Autodesk Fusion 360 part; units mm, degrees
note: some values were not read from the file. Set by a fixed rule: which sketch regions a step uses.
(part 8 of 15)
  line L6133 (281.912, -140.435) -> (281.972, -140.711)
  line L6134 (55.3535, -142.69) -> (55.0989, -142.813)
  line L6135 (56.3211, -141.359) -> (56.2444, -141.631)
  line L6136 (274.039, -141.862) -> (274.06, -141.678)
  line L6137 (56.1301, -141.889) -> (55.9807, -142.129)
  line L6138 (52.4255, -141.451) -> (52.3747, -141.173)
  line L6139 (52.6411, -141.971) -> (52.5149, -141.719)
  line L6140 (275.765, -142.423) -> (275.644, -142.563)
  line L6141 (52.5666, -140.073) -> (52.7085, -139.829)
  line L6142 (53.8349, -139.024) -> (54.112, -138.969)
  line L6143 (53.4546, -142.735) -> (53.2126, -142.589)
  line L6144 (56.3427, -140.671) -> (56.3626, -140.953)
  line L6145 (275.644, -142.563) -> (275.498, -142.677)
  line L6146 (275.52, -141.088) -> (275.663, -141.206)
  line L6147 (274.785, -142.803) -> (274.609, -142.746)
  line L6148 (52.4605, -140.335) -> (52.5666, -140.073)
  line L6149 (274.609, -142.746) -> (274.447, -142.655)
  line L6150 (274.447, -142.655) -> (274.306, -142.535)
  line L6151 (53.2126, -142.589) -> (52.9935, -142.411)
  line L6152 (56.2832, -140.395) -> (56.3427, -140.671)
  line L6153 (274.055, -142.047) -> (274.039, -141.862)
  line L6154 (56.3626, -140.953) -> (56.3587, -141.079)
  line L6155 (274.191, -142.39) -> (274.106, -142.225)
  line L6156 (275.18, -140.945) -> (275.357, -141)
  line L6157 (53.7148, -142.845) -> (53.4546, -142.735)
  line L6158 (275.939, -141.875) -> (275.939, -141.902)
  line L6159 (275.663, -141.206) -> (275.78, -141.35)
  line L6160 (275.857, -142.262) -> (275.765, -142.423)
  line L6161 (54.112, -138.969) -> (54.394, -138.953)
  line L6162 (275.357, -141) -> (275.52, -141.088)
  line L6163 (275.915, -142.086) -> (275.857, -142.262)
  line L6164 (52.8018, -142.204) -> (52.6411, -141.971)
  line L6165 (54.5508, -142.944) -> (54.2684, -142.951)
  line L6166 (53.5683, -139.118) -> (53.8349, -139.024)
  line L6167 (275.333, -142.761) -> (275.154, -142.811)
  line L6168 (54.394, -138.953) -> (54.6755, -138.978)
  line L6169 (55.7989, -142.345) -> (55.5884, -142.533)
  line L6170 (53.9879, -142.918) -> (53.7148, -142.845)
  line L6171 (56.1854, -140.13) -> (56.2832, -140.395)
  line L6172 (54.8295, -142.898) -> (54.5508, -142.944)
  line L6173 (275.78, -141.35) -> (275.867, -141.513)
  line L6174 (275.498, -142.677) -> (275.333, -142.761)
  line L6175 (275.921, -141.691) -> (275.939, -141.875)
  line L6176 (52.8834, -139.607) -> (53.0878, -139.412)
  line L6177 (53.0878, -139.412) -> (53.3176, -139.248)
  line L6178 (275.154, -142.811) -> (274.969, -142.825)
  line L6179 (274.106, -142.225) -> (274.055, -142.047)
  line L6180 (54.2684, -142.951) -> (53.9879, -142.918)
  line L6181 (59.1614, -142.763) -> (58.9851, -142.706)
  line L6182 (52.3636, -140.89) -> (52.3924, -140.609)
  line L6183 (52.3924, -140.609) -> (52.4605, -140.335)
  line L6184 (52.7085, -139.829) -> (52.8834, -139.607)
  line L6185 (53.3176, -139.248) -> (53.5683, -139.118)
  line L6186 (275.867, -141.513) -> (275.921, -141.691)
  line L6187 (55.0989, -142.813) -> (54.8295, -142.898)
  line L6188 (274.969, -142.825) -> (274.785, -142.803)
  line L6189 (274.306, -142.535) -> (274.191, -142.39)
  line L6190 (274.06, -141.678) -> (274.116, -141.501)
  line L6191 (52.9935, -142.411) -> (52.8018, -142.204)
  line L6192 (55.9807, -142.129) -> (55.7989, -142.345)
  line L6193 (275.939, -141.902) -> (275.915, -142.086)
  line L6194 (56.2444, -141.631) -> (56.1301, -141.889)
  line L6195 (52.3747, -141.173) -> (52.3636, -140.89)
  line L6196 (56.3587, -141.079) -> (56.3211, -141.359)
  line L6197 (55.5884, -142.533) -> (55.3535, -142.69)
  line L6198 (58.4155, -141.822) -> (58.4362, -141.638)
  line L6199 (60.1417, -142.383) -> (60.0206, -142.523)
  line L6200 (274.116, -141.501) -> (274.205, -141.339)
  line L6201 (60.2918, -142.046) -> (60.2333, -142.222)
  line L6202 (59.5565, -140.905) -> (59.7336, -140.96)
  line L6203 (274.324, -141.197) -> (274.469, -141.08)
  line L6204 (60.3154, -141.835) -> (60.3151, -141.862)
  line L6205 (59.3455, -142.785) -> (59.1614, -142.763)
  line L6206 (58.8233, -142.615) -> (58.6821, -142.495)
  line L6207 (60.1567, -141.31) -> (60.2438, -141.473)
  line L6208 (274.996, -140.925) -> (275.18, -140.945)
  line L6209 (58.9851, -142.706) -> (58.8233, -142.615)
  line L6210 (60.2333, -142.222) -> (60.1417, -142.383)
  line L6211 (59.8745, -142.637) -> (59.709, -142.721)
  line L6212 (274.469, -141.08) -> (274.633, -140.995)
  line L6213 (58.6821, -142.495) -> (58.5669, -142.35)
  line L6214 (60.2973, -141.651) -> (60.3154, -141.835)
  line L6215 (60.0206, -142.523) -> (59.8745, -142.637)
  line L6216 (274.811, -140.942) -> (274.996, -140.925)
  line L6217 (60.0395, -141.166) -> (60.1567, -141.31)
  line L6218 (59.709, -142.721) -> (59.5304, -142.771)
  line L6219 (59.7336, -140.96) -> (59.8967, -141.048)
  line L6220 (59.5304, -142.771) -> (59.3455, -142.785)
  line L6221 (60.2438, -141.473) -> (60.2973, -141.651)
  line L6222 (274.205, -141.339) -> (274.324, -141.197)
  line L6223 (58.4822, -142.185) -> (58.431, -142.007)
  line L6224 (58.5669, -142.35) -> (58.4822, -142.185)
  line L6225 (274.633, -140.995) -> (274.811, -140.942)
  line L6226 (300.674, -141.829) -> (300.463, -142.017)
  line L6227 (300.229, -142.174) -> (299.974, -142.296)
  line L6228 (301.005, -141.373) -> (300.856, -141.612)
  line L6229 (300.463, -142.017) -> (300.229, -142.174)
  line L6230 (299.705, -142.382) -> (299.426, -142.428)
  line L6231 (299.426, -142.428) -> (299.143, -142.435)
  line L6232 (301.158, -139.879) -> (301.218, -140.155)
  line L6233 (59.8967, -141.048) -> (60.0395, -141.166)
  line L6234 (58.8453, -141.04) -> (59.0096, -140.954)
  line L6235 (58.431, -142.007) -> (58.4155, -141.822)
  line L6236 (60.3151, -141.862) -> (60.2918, -142.046)
  line L6237 (300.926, -139.365) -> (301.06, -139.614)
  line L6238 (58.5816, -141.299) -> (58.7008, -141.157)
  line L6239 (301.234, -140.562) -> (301.196, -140.842)
  line L6240 (59.1874, -140.902) -> (59.3721, -140.885)
  line L6241 (59.3721, -140.885) -> (59.5565, -140.905)
  line L6242 (300.758, -139.138) -> (300.926, -139.365)
  line L6243 (300.56, -138.937) -> (300.758, -139.138)
  line L6244 (300.336, -138.765) -> (300.56, -138.937)
  line L6245 (301.06, -139.614) -> (301.158, -139.879)
  line L6246 (299.143, -142.435) -> (298.863, -142.401)
  line L6247 (298.863, -142.401) -> (298.59, -142.329)
  line L6248 (300.856, -141.612) -> (300.674, -141.829)
  line L6249 (59.0096, -140.954) -> (59.1874, -140.902)
  line L6250 (301.218, -140.155) -> (301.238, -140.437)
  line L6251 (35.7049, -138.485) -> (35.9684, -138.587)
  line L6252 (58.4923, -141.461) -> (58.5816, -141.299)
  line L6253 (58.4362, -141.638) -> (58.4923, -141.461)
  line L6254 (300.089, -138.627) -> (300.336, -138.765)
  line L6255 (299.826, -138.525) -> (300.089, -138.627)
  line L6256 (301.238, -140.437) -> (301.234, -140.562)
  line L6257 (58.7008, -141.157) -> (58.8453, -141.04)
  line L6258 (37.1169, -140.397) -> (37.1129, -140.522)
  line L6259 (299.551, -138.461) -> (299.826, -138.525)
  line L6260 (299.974, -142.296) -> (299.705, -142.382)
  line L6261 (301.196, -140.842) -> (301.119, -141.114)
  line L6262 (301.119, -141.114) -> (301.005, -141.373)
  line L6263 (298.33, -142.219) -> (298.088, -142.073)
  line L6264 (298.088, -142.073) -> (297.869, -141.895)
  line L6265 (36.2149, -138.725) -> (36.4395, -138.896)
  line L6266 (297.267, -140.093) -> (297.336, -139.819)
  line L6267 (298.193, -138.731) -> (298.443, -138.601)
  line L6268 (297.336, -139.819) -> (297.442, -139.557)
  line L6269 (297.963, -138.896) -> (298.193, -138.731)
  line L6270 (298.59, -142.329) -> (298.33, -142.219)
  line L6271 (36.4395, -138.896) -> (36.6377, -139.098)
  line L6272 (297.869, -141.895) -> (297.677, -141.687)
  line L6273 (298.987, -138.453) -> (299.269, -138.437)
  line L6274 (297.239, -140.374) -> (297.267, -140.093)
  line L6275 (297.25, -140.656) -> (297.239, -140.374)
  line L6276 (36.6377, -139.098) -> (36.8055, -139.325)
  line L6277 (35.9684, -138.587) -> (36.2149, -138.725)
  line L6278 (36.9397, -139.574) -> (37.0374, -139.839)
  line L6279 (297.583, -139.313) -> (297.758, -139.091)
  line L6280 (36.8055, -139.325) -> (36.9397, -139.574)
  line L6281 (298.71, -138.508) -> (298.987, -138.453)
  line L6282 (37.0374, -139.839) -> (37.0969, -140.115)
  line L6283 (35.4297, -138.421) -> (35.7049, -138.485)
  line L6284 (297.3, -140.934) -> (297.25, -140.656)
  line L6285 (322.128, -135.872) -> (322.217, -135.71)
  line L6286 (11.1494, -137.134) -> (10.9731, -137.077)
  line L6287 (12.2854, -136.022) -> (12.3034, -136.207)
  line L6288 (11.5184, -137.142) -> (11.3336, -137.156)
  line L6289 (322.217, -135.71) -> (322.336, -135.568)
  line L6290 (11.5445, -135.276) -> (11.7216, -135.331)
  line L6291 (322.645, -135.366) -> (322.823, -135.313)
  line L6292 (259.789, -140.345) -> (260.04, -140.214)
  line L6293 (260.584, -140.066) -> (260.866, -140.05)
  line L6294 (12.1447, -135.681) -> (12.2318, -135.845)
  line L6295 (12.3031, -136.233) -> (12.2798, -136.417)
  line L6296 (322.051, -136.233) -> (322.072, -136.049)
  line L6297 (10.9731, -137.077) -> (10.8113, -136.987)
  line L6298 (12.0086, -136.895) -> (11.8625, -137.009)
  line L6299 (10.8113, -136.987) -> (10.6701, -136.866)
  line L6300 (322.072, -136.049) -> (322.128, -135.872)
  line L6301 (11.8847, -135.419) -> (12.0275, -135.537)
  line L6302 (10.6701, -136.866) -> (10.5549, -136.721)
  line L6303 (12.2318, -135.845) -> (12.2854, -136.022)
  line L6304 (11.7216, -135.331) -> (11.8847, -135.419)
  line L6305 (12.0275, -135.537) -> (12.1447, -135.681)
  line L6306 (322.067, -136.418) -> (322.051, -136.233)
  line L6307 (140.338, -80.776) -> (140.444, -80.5142)
  line L6308 (227.517, -73.5849) -> (227.391, -73.3322)
  line L6309 (140.27, -81.0502) -> (140.338, -80.776)
  line L6310 (142.271, -79.3943) -> (142.553, -79.4187)
  line L6311 (228.331, -74.3489) -> (228.089, -74.2032)
  line L6312 (140.871, -82.852) -> (140.679, -82.6445)
  line L6313 (140.965, -79.853) -> (141.195, -79.6888)
  line L6314 (227.269, -72.223) -> (227.337, -71.9488)
  line L6315 (230.23, -74.3041) -> (229.975, -74.4264)
  line L6316 (228.591, -74.459) -> (228.331, -74.3489)
  line L6317 (228.444, -70.7313) -> (228.711, -70.6377)
  line L6318 (227.964, -71.0258) -> (228.194, -70.8616)
  line L6319 (142.707, -83.3388) -> (142.428, -83.3852)
  line L6320 (227.678, -73.8173) -> (227.517, -73.5849)
  line L6321 (141.09, -83.0304) -> (140.871, -82.852)
  line L6322 (187.786, -81.6469) -> (187.903, -81.7905)
  line L6323 (206.499, -137.614) -> (206.358, -137.494)
  line L6324 (206.257, -136.297) -> (206.377, -136.155)
  line L6325 (207.409, -135.958) -> (207.573, -136.046)
  line L6326 (207.55, -137.636) -> (207.385, -137.719)
  line L6327 (206.243, -137.348) -> (206.158, -137.183)
  line L6328 (207.573, -136.046) -> (207.715, -136.164)
  line L6329 (207.968, -137.044) -> (207.909, -137.22)
  line L6330 (206.112, -136.636) -> (206.168, -136.46)
  line L6331 (206.661, -137.704) -> (206.499, -137.614)
  line L6332 (206.377, -136.155) -> (206.521, -136.039)
  line L6333 (206.168, -136.46) -> (206.257, -136.297)
  line L6334 (206.837, -137.762) -> (206.661, -137.704)
  line L6335 (21.1811, -137.038) -> (21.3657, -137.021)
  line L6336 (206.358, -137.494) -> (206.243, -137.348)
  line L6337 (207.833, -136.308) -> (207.92, -136.472)
  line L6338 (21.3657, -137.021) -> (21.5501, -137.04)
  line L6339 (206.107, -137.005) -> (206.091, -136.82)
  line L6340 (206.521, -136.039) -> (206.685, -135.953)
  line L6341 (207.232, -135.903) -> (207.409, -135.958)
  line L6342 (206.091, -136.82) -> (206.112, -136.636)
  line L6343 (207.385, -137.719) -> (207.206, -137.769)
  line L6344 (207.715, -136.164) -> (207.833, -136.308)
  line L6345 (206.158, -137.183) -> (206.107, -137.005)
  line L6346 (126.363, -136.78) -> (126.384, -136.596)
  line L6347 (207.818, -137.381) -> (207.696, -137.522)
  line L6348 (127.968, -137.482) -> (127.822, -137.596)
  line L6349 (126.63, -137.454) -> (126.515, -137.308)
  line L6350 (128.263, -136.794) -> (128.263, -136.82)
  line L6351 (127.681, -135.918) -> (127.844, -136.006)
  line L6352 (128.24, -137.004) -> (128.181, -137.18)
  line L6353 (126.771, -137.574) -> (126.63, -137.454)
  line L6354 (128.089, -137.341) -> (127.968, -137.482)
  line L6355 (207.021, -137.784) -> (206.837, -137.762)
  line L6356 (207.92, -136.472) -> (207.973, -136.649)
  line L6357 (207.206, -137.769) -> (207.021, -137.784)
  line L6358 (126.933, -137.664) -> (126.771, -137.574)
  line L6359 (128.192, -136.432) -> (128.245, -136.609)
  line L6360 (126.529, -136.257) -> (126.649, -136.115)
  line L6361 (126.44, -136.419) -> (126.529, -136.257)
  line L6362 (206.685, -135.953) -> (206.863, -135.901)
  line L6363 (127.504, -135.863) -> (127.681, -135.918)
  line L6364 (127.293, -137.743) -> (127.109, -137.722)
  line L6365 (126.379, -136.965) -> (126.363, -136.78)
  line L6366 (126.43, -137.143) -> (126.379, -136.965)
  line L6367 (127.844, -136.006) -> (127.987, -136.124)
  line L6368 (126.515, -137.308) -> (126.43, -137.143)
  line L6369 (207.973, -136.649) -> (207.991, -136.834)
  line L6370 (126.384, -136.596) -> (126.44, -136.419)
  line L6371 (127.109, -137.722) -> (126.933, -137.664)
  line L6372 (127.987, -136.124) -> (128.104, -136.268)
  line L6373 (207.991, -136.834) -> (207.991, -136.86)
  line L6374 (206.863, -135.901) -> (207.048, -135.884)
  line L6375 (128.245, -136.609) -> (128.263, -136.794)
  line L6376 (128.104, -136.268) -> (128.192, -136.432)
  line L6377 (127.822, -137.596) -> (127.657, -137.679)
  line L6378 (323.792, -135.721) -> (323.879, -135.885)
  line L6379 (323.879, -135.885) -> (323.933, -136.062)
  line L6380 (126.793, -135.999) -> (126.957, -135.913)
  line L6381 (127.32, -135.844) -> (127.504, -135.863)
  line L6382 (322.318, -136.907) -> (322.203, -136.761)
  line L6383 (323.675, -135.577) -> (323.792, -135.721)
  line L6384 (323.166, -137.182) -> (322.981, -137.196)
  line L6385 (323.192, -135.316) -> (323.369, -135.371)
  line L6386 (323.51, -137.049) -> (323.345, -137.132)
  line L6387 (323.369, -135.371) -> (323.532, -135.459)
  line L6388 (323.951, -136.247) -> (323.951, -136.273)
  line L6389 (127.657, -137.679) -> (127.478, -137.729)
  line L6390 (127.478, -137.729) -> (127.293, -137.743)
  line L6391 (128.181, -137.18) -> (128.089, -137.341)
  line L6392 (323.777, -136.794) -> (323.656, -136.935)
  line L6393 (126.649, -136.115) -> (126.793, -135.999)
  line L6394 (323.345, -137.132) -> (323.166, -137.182)
  line L6395 (323.933, -136.062) -> (323.951, -136.247)
  line L6396 (323.927, -136.457) -> (323.869, -136.633)
  line L6397 (128.263, -136.82) -> (128.24, -137.004)
  line L6398 (322.981, -137.196) -> (322.797, -137.174)
  line L6399 (322.797, -137.174) -> (322.621, -137.117)
  line L6400 (323.951, -136.273) -> (323.927, -136.457)
  line L6401 (322.621, -137.117) -> (322.459, -137.027)
  line L6402 (323.532, -135.459) -> (323.675, -135.577)
  line L6403 (323.869, -136.633) -> (323.777, -136.794)
  line L6404 (126.957, -135.913) -> (127.135, -135.861)
  line L6405 (207.048, -135.884) -> (207.232, -135.903)
  line L6406 (323.656, -136.935) -> (323.51, -137.049)
  line L6407 (127.135, -135.861) -> (127.32, -135.844)
  line L6408 (322.459, -137.027) -> (322.318, -136.907)
  line L6409 (322.203, -136.761) -> (322.118, -136.596)
  line L6410 (221.651, -132.598) -> (221.897, -132.736)
  line L6411 (221.112, -132.433) -> (221.387, -132.496)
  line L6412 (10.4191, -136.378) -> (10.4035, -136.193)
  line L6413 (222.488, -133.336) -> (222.622, -133.585)
  line L6414 (11.1754, -135.273) -> (11.3601, -135.257)
  line L6415 (10.9976, -135.326) -> (11.1754, -135.273)
  line L6416 (10.4242, -136.009) -> (10.4803, -135.832)
  line L6417 (222.622, -133.585) -> (222.72, -133.85)
  line L6418 (222.681, -135.085) -> (222.567, -135.344)
  line L6419 (222.025, -135.988) -> (221.79, -136.145)
  line L6420 (222.799, -134.408) -> (222.795, -134.533)
  line L6421 (10.4035, -136.193) -> (10.4242, -136.009)
  line L6422 (10.4702, -136.556) -> (10.4191, -136.378)
  line L6423 (222.235, -135.8) -> (222.025, -135.988)
  line L6424 (11.3601, -135.257) -> (11.5445, -135.276)
  line L6425 (10.6888, -135.528) -> (10.8333, -135.412)
  line L6426 (221.535, -136.267) -> (221.266, -136.353)
  line L6427 (222.32, -133.109) -> (222.488, -133.336)
  line L6428 (10.4803, -135.832) -> (10.5696, -135.67)
  line L6429 (222.417, -135.583) -> (222.235, -135.8)
  line L6430 (221.897, -132.736) -> (222.122, -132.908)
  line L6431 (222.758, -134.813) -> (222.681, -135.085)
  line L6432 (222.72, -133.85) -> (222.779, -134.126)
  line L6433 (221.79, -136.145) -> (221.535, -136.267)
  line L6434 (222.567, -135.344) -> (222.417, -135.583)
  line L6435 (222.122, -132.908) -> (222.32, -133.109)
  line L6436 (10.5696, -135.67) -> (10.6888, -135.528)
  line L6437 (221.387, -132.496) -> (221.651, -132.598)
  line L6438 (10.8333, -135.412) -> (10.9976, -135.326)
  line L6439 (10.5549, -136.721) -> (10.4702, -136.556)
  line L6440 (222.779, -134.126) -> (222.799, -134.408)
  line L6441 (222.795, -134.533) -> (222.758, -134.813)
  line L6442 (219.649, -136.044) -> (219.43, -135.866)
  line L6443 (221.266, -136.353) -> (220.987, -136.399)
  line L6444 (114.143, -132.456) -> (114.407, -132.558)
  line L6445 (220.705, -136.406) -> (220.424, -136.372)
  line L6446 (219.891, -136.19) -> (219.649, -136.044)
  line L6447 (220.987, -136.399) -> (220.705, -136.406)
  line L6448 (218.811, -134.627) -> (218.8, -134.345)
  line L6449 (218.862, -134.905) -> (218.811, -134.627)
  line L6450 (113.868, -132.392) -> (114.143, -132.456)
  line L6451 (218.829, -134.064) -> (218.897, -133.79)
  line L6452 (115.076, -133.069) -> (115.244, -133.296)
  line L6453 (114.653, -132.696) -> (114.878, -132.868)
  line L6454 (219.754, -132.703) -> (220.005, -132.572)
  line L6455 (220.831, -132.408) -> (221.112, -132.433)
  line L6456 (220.548, -132.424) -> (220.831, -132.408)
  line L6457 (218.897, -133.79) -> (219.003, -133.528)
  line L6458 (114.878, -132.868) -> (115.076, -133.069)
  line L6459 (219.524, -132.867) -> (219.754, -132.703)
  line L6460 (115.244, -133.296) -> (115.378, -133.545)
  line L6461 (220.151, -136.3) -> (219.891, -136.19)
  line L6462 (218.8, -134.345) -> (218.829, -134.064)
  line L6463 (220.271, -132.479) -> (220.548, -132.424)
  line L6464 (114.407, -132.558) -> (114.653, -132.696)
  line L6465 (219.145, -133.284) -> (219.32, -133.062)
  line L6466 (112.908, -136.26) -> (112.647, -136.15)
  line L6467 (219.078, -135.426) -> (218.951, -135.173)
  line L6468 (111.708, -135.133) -> (111.618, -134.865)
  line L6469 (111.759, -133.488) -> (111.901, -133.244)
  line L6470 (220.424, -136.372) -> (220.151, -136.3)
  line L6471 (111.653, -133.75) -> (111.759, -133.488)
  line L6472 (112.076, -133.022) -> (112.281, -132.827)
  line L6473 (112.186, -135.826) -> (111.995, -135.618)
  line L6474 (115.535, -134.086) -> (115.555, -134.368)
  line L6475 (115.378, -133.545) -> (115.476, -133.81)
  line L6476 (115.476, -133.81) -> (115.535, -134.086)
  line L6477 (112.405, -136.004) -> (112.186, -135.826)
  line L6478 (111.567, -134.587) -> (111.556, -134.305)
  line L6479 (219.43, -135.866) -> (219.238, -135.658)
  line L6480 (112.647, -136.15) -> (112.405, -136.004)
  line L6481 (111.585, -134.024) -> (111.653, -133.75)
  line L6482 (219.238, -135.658) -> (219.078, -135.426)
  line L6483 (111.901, -133.244) -> (112.076, -133.022)
  line L6484 (219.32, -133.062) -> (219.524, -132.867)
  line L6485 (115.555, -134.368) -> (115.551, -134.493)
  line L6486 (218.951, -135.173) -> (218.862, -134.905)
  line L6487 (219.003, -133.528) -> (219.145, -133.284)
  line L6488 (115.437, -135.045) -> (115.323, -135.304)
  line L6489 (220.005, -132.572) -> (220.271, -132.479)
  line L6490 (115.173, -135.543) -> (114.992, -135.76)
  line L6491 (114.546, -136.105) -> (114.292, -136.227)
  line L6492 (114.781, -135.948) -> (114.546, -136.105)
  line L6493 (113.181, -136.332) -> (112.908, -136.26)
  line L6494 (113.461, -136.366) -> (113.181, -136.332)
  line L6495 (111.556, -134.305) -> (111.585, -134.024)
  line L6496 (115.514, -134.773) -> (115.437, -135.045)
  line L6497 (111.834, -135.386) -> (111.708, -135.133)
  line L6498 (115.323, -135.304) -> (115.173, -135.543)
  line L6499 (115.551, -134.493) -> (115.514, -134.773)
  line L6500 (113.744, -136.359) -> (113.461, -136.366)
  line L6501 (114.022, -136.313) -> (113.744, -136.359)
  line L6502 (114.292, -136.227) -> (114.022, -136.313)
  line L6503 (111.995, -135.618) -> (111.834, -135.386)
  line L6504 (114.992, -135.76) -> (114.781, -135.948)
  line L6505 (111.618, -134.865) -> (111.567, -134.587)
  line L6506 (216.588, -134.764) -> (216.675, -134.928)
  line L6507 (215.776, -136.24) -> (215.592, -136.218)
  line L6508 (113.028, -132.439) -> (113.305, -132.384)
  line L6509 (215.113, -135.95) -> (214.998, -135.805)
  line L6510 (216.573, -135.838) -> (216.451, -135.978)
  line L6511 (214.913, -135.64) -> (214.862, -135.462)
  line L6512 (214.846, -135.277) -> (214.867, -135.093)
  line L6513 (215.254, -136.07) -> (215.113, -135.95)
  line L6514 (216.327, -134.502) -> (216.47, -134.621)
  line L6515 (215.987, -134.359) -> (216.164, -134.414)
  line L6516 (216.664, -135.676) -> (216.573, -135.838)
  line L6517 (216.728, -135.105) -> (216.746, -135.29)
  line L6518 (216.47, -134.621) -> (216.588, -134.764)
  line L6519 (215.592, -136.218) -> (215.416, -136.161)
  line L6520 (214.862, -135.462) -> (214.846, -135.277)
  line L6521 (215.961, -136.226) -> (215.776, -136.24)
  line L6522 (113.587, -132.368) -> (113.868, -132.392)
  line L6523 (216.675, -134.928) -> (216.728, -135.105)
  line L6524 (216.451, -135.978) -> (216.305, -136.092)
  line L6525 (112.281, -132.827) -> (112.51, -132.663)
  line L6526 (215.012, -134.753) -> (215.132, -134.611)
  line L6527 (215.803, -134.34) -> (215.987, -134.359)
  line L6528 (119.35, -134.724) -> (119.437, -134.888)
  line L6529 (215.416, -136.161) -> (215.254, -136.07)
  line L6530 (118.749, -134.319) -> (118.926, -134.374)
  line L6531 (118.538, -136.2) -> (118.354, -136.178)
  line L6532 (117.624, -135.421) -> (117.608, -135.237)
  line L6533 (113.305, -132.384) -> (113.587, -132.368)
  line L6534 (216.305, -136.092) -> (216.14, -136.176)
  line L6535 (214.998, -135.805) -> (214.913, -135.64)
  line L6536 (215.44, -134.409) -> (215.618, -134.357)
  line L6537 (119.437, -134.888) -> (119.49, -135.065)
  line L6538 (214.923, -134.916) -> (215.012, -134.753)
  line L6539 (216.14, -136.176) -> (215.961, -136.226)
  line L6540 (215.618, -134.357) -> (215.803, -134.34)
  line L6541 (117.875, -135.91) -> (117.76, -135.765)
  line L6542 (117.675, -135.6) -> (117.624, -135.421)
  line L6543 (216.746, -135.317) -> (216.723, -135.5)
  line L6544 (216.723, -135.5) -> (216.664, -135.676)
  line L6545 (118.723, -136.186) -> (118.538, -136.2)
  line L6546 (216.746, -135.29) -> (216.746, -135.317)
  line L6547 (216.164, -134.414) -> (216.327, -134.502)
  line L6548 (112.51, -132.663) -> (112.761, -132.532)
  line L6549 (112.761, -132.532) -> (113.028, -132.439)
  line L6550 (119.232, -134.581) -> (119.35, -134.724)
  line L6551 (214.867, -135.093) -> (214.923, -134.916)
  line L6552 (118.926, -134.374) -> (119.089, -134.462)
  line L6553 (118.016, -136.03) -> (117.875, -135.91)
  line L6554 (118.902, -136.136) -> (118.723, -136.186)
  line L6555 (118.178, -136.12) -> (118.016, -136.03)
  line L6556 (119.49, -135.065) -> (119.508, -135.25)
  line L6557 (119.213, -135.938) -> (119.067, -136.052)
  line L6558 (215.132, -134.611) -> (215.276, -134.495)
  line L6559 (119.508, -135.25) -> (119.508, -135.276)
  line L6560 (119.485, -135.46) -> (119.426, -135.636)
  line L6561 (117.608, -135.237) -> (117.629, -135.052)
  line L6562 (119.426, -135.636) -> (119.335, -135.798)
  line L6563 (119.508, -135.276) -> (119.485, -135.46)
  line L6564 (119.067, -136.052) -> (118.902, -136.136)
  line L6565 (119.089, -134.462) -> (119.232, -134.581)
  line L6566 (215.276, -134.495) -> (215.44, -134.409)
  line L6567 (119.335, -135.798) -> (119.213, -135.938)
  line L6568 (225.598, -134.454) -> (225.422, -134.396)
  line L6569 (226.728, -133.736) -> (226.67, -133.912)
  line L6570 (225.003, -134.04) -> (224.919, -133.875)
  line L6571 (226.476, -132.856) -> (226.593, -133)
  line L6572 (118.038, -134.455) -> (118.202, -134.369)
  line L6573 (117.685, -134.876) -> (117.774, -134.713)
  line L6574 (226.311, -134.328) -> (226.145, -134.411)
  line L6575 (225.782, -134.476) -> (225.598, -134.454)
  line L6576 (117.76, -135.765) -> (117.675, -135.6)
  line L6577 (225.967, -134.461) -> (225.782, -134.476)
  line L6578 (226.593, -133) -> (226.68, -133.164)
  line L6579 (117.629, -135.052) -> (117.685, -134.876)
  line L6580 (226.17, -132.65) -> (226.333, -132.738)
  line L6581 (226.752, -133.526) -> (226.752, -133.552)
  line L6582 (226.457, -134.214) -> (226.311, -134.328)
  line L6583 (225.422, -134.396) -> (225.26, -134.306)
  line L6584 (224.919, -133.875) -> (224.868, -133.697)
  line L6585 (226.145, -134.411) -> (225.967, -134.461)
  line L6586 (224.868, -133.697) -> (224.852, -133.512)
  line L6587 (225.119, -134.186) -> (225.003, -134.04)
  line L6588 (226.752, -133.552) -> (226.728, -133.736)
  line L6589 (226.67, -133.912) -> (226.578, -134.073)
  line L6590 (226.333, -132.738) -> (226.476, -132.856)
  line L6591 (118.38, -134.317) -> (118.565, -134.3)
  line L6592 (225.993, -132.595) -> (226.17, -132.65)
  line L6593 (118.565, -134.3) -> (118.749, -134.319)
  line L6594 (225.26, -134.306) -> (225.119, -134.186)
  line L6595 (117.774, -134.713) -> (117.894, -134.571)
  line L6596 (117.894, -134.571) -> (118.038, -134.455)
  line L6597 (226.734, -133.341) -> (226.752, -133.526)
  line L6598 (118.202, -134.369) -> (118.38, -134.317)
  line L6599 (118.354, -136.178) -> (118.178, -136.12)
  line L6600 (226.578, -134.073) -> (226.457, -134.214)
  line L6601 (108.01, -134.266) -> (107.869, -134.146)
  line L6602 (109.502, -133.512) -> (109.479, -133.696)
  line L6603 (109.208, -134.174) -> (109.062, -134.288)
  line L6604 (224.929, -133.152) -> (225.018, -132.989)
  line L6605 (225.624, -132.593) -> (225.809, -132.576)
  line L6606 (109.479, -133.696) -> (109.42, -133.872)
  line L6607 (108.349, -134.414) -> (108.172, -134.356)
  line L6608 (107.869, -134.146) -> (107.754, -134)
  line L6609 (224.852, -133.512) -> (224.873, -133.328)
  line L6610 (109.062, -134.288) -> (108.896, -134.371)
  line L6611 (107.669, -133.835) -> (107.618, -133.657)
  line L6612 (109.485, -133.301) -> (109.503, -133.486)
  line L6613 (108.744, -132.555) -> (108.921, -132.61)
  line L6614 (225.137, -132.847) -> (225.282, -132.731)
  line L6615 (108.921, -132.61) -> (109.084, -132.698)
  line L6616 (109.344, -132.96) -> (109.431, -133.124)
  line L6617 (109.329, -134.033) -> (109.208, -134.174)
  line L6618 (225.446, -132.645) -> (225.624, -132.593)
  line L6619 (107.754, -134) -> (107.669, -133.835)
  line L6620 (108.718, -134.421) -> (108.533, -134.435)
  line L6621 (225.282, -132.731) -> (225.446, -132.645)
  line L6622 (225.018, -132.989) -> (225.137, -132.847)
  line L6623 (224.873, -133.328) -> (224.929, -133.152)
  line L6624 (226.68, -133.164) -> (226.734, -133.341)
  line L6625 (109.227, -132.816) -> (109.344, -132.96)
  line L6626 (109.503, -133.486) -> (109.502, -133.512)
  line L6627 (108.172, -134.356) -> (108.01, -134.266)
  line L6628 (225.809, -132.576) -> (225.993, -132.595)
  line L6629 (312.331, -137.332) -> (312.475, -137.216)
  line L6630 (312.817, -137.078) -> (313.002, -137.061)
  line L6631 (312.64, -137.13) -> (312.817, -137.078)
  line L6632 (313.651, -138.699) -> (313.504, -138.813)
  line L6633 (313.927, -137.826) -> (313.945, -138.011)
  line L6634 (313.339, -138.897) -> (313.16, -138.946)
  line L6635 (312.046, -137.998) -> (312.066, -137.813)
  line L6636 (313.787, -137.485) -> (313.874, -137.649)
  line L6637 (313.527, -137.223) -> (313.67, -137.341)
  line L6638 (312.212, -137.474) -> (312.331, -137.332)
  line L6639 (313.874, -137.649) -> (313.927, -137.826)
  line L6640 (313.504, -138.813) -> (313.339, -138.897)
  line L6641 (313.16, -138.946) -> (312.976, -138.961)
  line L6642 (312.197, -138.526) -> (312.112, -138.361)
  line L6643 (312.453, -138.791) -> (312.312, -138.671)
  line L6644 (312.312, -138.671) -> (312.197, -138.526)
  line L6645 (21.5501, -137.04) -> (21.7272, -137.095)
  line L6646 (20.8169, -138.751) -> (20.6757, -138.631)
  line L6647 (22.2374, -137.609) -> (22.291, -137.786)
  line L6648 (21.3392, -138.921) -> (21.1551, -138.899)
  line L6649 (22.1504, -137.445) -> (22.2374, -137.609)
  line L6650 (312.112, -138.361) -> (312.061, -138.182)
  line L6651 (21.7272, -137.095) -> (21.8903, -137.183)
  line L6652 (20.4299, -137.773) -> (20.4859, -137.597)
  line L6653 (20.4758, -138.321) -> (20.4247, -138.142)
  line L6654 (20.4859, -137.597) -> (20.5752, -137.434)
  line L6655 (20.8389, -137.176) -> (21.0032, -137.09)
  line L6656 (21.0032, -137.09) -> (21.1811, -137.038)
  line L6657 (20.5606, -138.485) -> (20.4758, -138.321)
  line L6658 (20.4092, -137.958) -> (20.4299, -137.773)
  line L6659 (20.6944, -137.292) -> (20.8389, -137.176)
  line L6660 (20.6757, -138.631) -> (20.5606, -138.485)
  line L6661 (20.5752, -137.434) -> (20.6944, -137.292)
  line L6662 (22.3091, -137.971) -> (22.3087, -137.997)
  line L6663 (22.0142, -138.659) -> (21.8681, -138.773)
  line L6664 (21.8903, -137.183) -> (22.0332, -137.301)
  line L6665 (22.291, -137.786) -> (22.3091, -137.971)
  line L6666 (22.2855, -138.181) -> (22.227, -138.357)
  line L6667 (21.1551, -138.899) -> (20.9788, -138.841)
  line L6668 (20.4247, -138.142) -> (20.4092, -137.958)
  line L6669 (22.1354, -138.518) -> (22.0142, -138.659)
  line L6670 (22.0332, -137.301) -> (22.1504, -137.445)
  line L6671 (21.8681, -138.773) -> (21.7026, -138.857)
  line L6672 (20.9788, -138.841) -> (20.8169, -138.751)
  line L6673 (22.3087, -137.997) -> (22.2855, -138.181)
  line L6674 (21.7026, -138.857) -> (21.5241, -138.906)
  line L6675 (22.227, -138.357) -> (22.1354, -138.518)
  line L6676 (21.5241, -138.906) -> (21.3392, -138.921)
  line L6677 (313.002, -137.061) -> (313.186, -137.08)
  line L6678 (207.696, -137.522) -> (207.55, -137.636)
  line L6679 (207.991, -136.86) -> (207.968, -137.044)
  line L6680 (207.909, -137.22) -> (207.818, -137.381)
  line L6681 (310.219, -118.463) -> (310.362, -118.581)
  line L6682 (18.6193, -116.623) -> (18.87, -116.493)
  line L6683 (310.566, -118.888) -> (310.619, -119.066)
  line L6684 (310.619, -119.066) -> (310.637, -119.25)
  line L6685 (310.637, -119.25) -> (310.637, -119.277)
  line L6686 (25.3412, -118.541) -> (25.4584, -118.685)
  line L6687 (25.6171, -119.21) -> (25.6167, -119.237)
  line L6688 (18.3894, -116.787) -> (18.6193, -116.623)
  line L6689 (309.509, -118.317) -> (309.694, -118.3)
  line L6690 (309.023, -118.572) -> (309.167, -118.455)
  line L6691 (25.4584, -118.685) -> (25.5454, -118.848)
  line L6692 (25.5454, -118.848) -> (25.599, -119.026)
  line L6693 (25.599, -119.026) -> (25.6171, -119.21)
  line L6694 (25.3222, -119.898) -> (25.1761, -120.012)
  line L6695 (308.814, -118.876) -> (308.904, -118.714)
  line L6696 (25.1761, -120.012) -> (25.0106, -120.096)
  line L6697 (18.185, -116.982) -> (18.3894, -116.787)
  line L6698 (25.4434, -119.758) -> (25.3222, -119.898)
  line L6699 (309.332, -118.369) -> (309.509, -118.317)
  line L6700 (25.0106, -120.096) -> (24.8321, -120.146)
  line L6701 (25.535, -119.597) -> (25.4434, -119.758)
  line L6702 (310.056, -118.375) -> (310.219, -118.463)
  line L6703 (309.878, -118.32) -> (310.056, -118.375)
  line L6704 (308.753, -119.422) -> (308.738, -119.237)
  line L6705 (25.0352, -118.334) -> (25.1983, -118.423)
  line L6706 (24.6472, -120.16) -> (24.4631, -120.138)
  line L6707 (24.8321, -120.146) -> (24.6472, -120.16)
  line L6708 (25.1983, -118.423) -> (25.3412, -118.541)
  line L6709 (25.6167, -119.237) -> (25.5935, -119.421)
  line L6710 (308.904, -118.714) -> (309.023, -118.572)
  line L6711 (25.5935, -119.421) -> (25.535, -119.597)
  line L6712 (24.4631, -120.138) -> (24.2868, -120.081)
  line L6713 (24.2868, -120.081) -> (24.1249, -119.99)
  line L6714 (309.167, -118.455) -> (309.332, -118.369)
  line L6715 (309.004, -119.91) -> (308.889, -119.765)
  line L6716 (308.889, -119.765) -> (308.804, -119.6)
  line L6717 (308.804, -119.6) -> (308.753, -119.422)
  line L6718 (196.743, -119.175) -> (196.731, -118.892)
  line L6719 (197.58, -120.592) -> (197.361, -120.413)
  line L6720 (32.4721, -120.741) -> (32.4928, -120.556)
  line L6721 (196.731, -118.892) -> (196.76, -118.611)
  line L6722 (196.828, -118.337) -> (196.934, -118.075)
  line L6723 (32.7387, -121.414) -> (32.6235, -121.269)
  line L6724 (197.823, -120.737) -> (197.58, -120.592)
  line L6725 (200.731, -118.955) -> (200.727, -119.081)
  line L6726 (197.009, -119.973) -> (196.883, -119.721)
  line L6727 (196.934, -118.075) -> (197.076, -117.831)
  line L6728 (197.076, -117.831) -> (197.251, -117.609)
  line L6729 (32.4876, -120.925) -> (32.4721, -120.741)
  line L6730 (33.0417, -121.625) -> (32.8799, -121.534)
  line L6731 (32.7574, -120.075) -> (32.9018, -119.959)
  line L6732 (32.8799, -121.534) -> (32.7387, -121.414)
  line L6733 (199.582, -117.146) -> (199.829, -117.284)
  line L6734 (196.883, -119.721) -> (196.793, -119.453)
  line L6735 (32.4928, -120.556) -> (32.5489, -120.38)
  line L6736 (197.251, -117.609) -> (197.456, -117.414)
  line L6737 (200.498, -119.891) -> (200.349, -120.131)
  line L6738 (198.083, -120.847) -> (197.823, -120.737)
  line L6739 (198.919, -120.946) -> (198.636, -120.953)
  line L6740 (200.612, -119.633) -> (200.498, -119.891)
  line L6741 (199.467, -120.815) -> (199.197, -120.9)
  line L6742 (199.721, -120.693) -> (199.467, -120.815)
  line L6743 (200.727, -119.081) -> (200.689, -119.361)
  line L6744 (200.349, -120.131) -> (200.167, -120.347)
  line L6745 (137.06, -120.307) -> (136.85, -120.496)
  line L6746 (137.506, -119.593) -> (137.392, -119.851)
  line L6747 (137.545, -118.357) -> (137.604, -118.633)
  line L6748 (197.361, -120.413) -> (197.17, -120.206)
  line L6749 (137.447, -118.092) -> (137.545, -118.357)
  line L6750 (197.686, -117.25) -> (197.936, -117.12)
  line L6751 (136.212, -117.004) -> (136.476, -117.106)
  line L6752 (198.636, -120.953) -> (198.356, -120.92)
  line L6753 (199.197, -120.9) -> (198.919, -120.946)
  line L6754 (196.76, -118.611) -> (196.828, -118.337)
  line L6755 (200.689, -119.361) -> (200.612, -119.633)
  line L6756 (134.716, -120.697) -> (134.474, -120.552)
  line L6757 (134.976, -120.807) -> (134.716, -120.697)
  line L6758 (197.936, -117.12) -> (198.203, -117.026)
  line L6759 (199.956, -120.536) -> (199.721, -120.693)
  line L6760 (197.17, -120.206) -> (197.009, -119.973)
  line L6761 (198.356, -120.92) -> (198.083, -120.847)
  line L6762 (197.456, -117.414) -> (197.686, -117.25)
  line L6763 (135.937, -116.94) -> (136.212, -117.004)
  line L6764 (200.167, -120.347) -> (199.956, -120.536)
  line L6765 (137.62, -119.041) -> (137.582, -119.321)
  line L6766 (196.793, -119.453) -> (196.743, -119.175)
  line L6767 (135.249, -120.88) -> (134.976, -120.807)
  line L6768 (134.474, -120.552) -> (134.255, -120.373)
  line L6769 (137.313, -117.844) -> (137.447, -118.092)
  line L6770 (134.063, -120.166) -> (133.903, -119.933)
  line L6771 (137.392, -119.851) -> (137.242, -120.091)
  line L6772 (134.255, -120.373) -> (134.063, -120.166)
  line L6773 (137.242, -120.091) -> (137.06, -120.307)
  line L6774 (137.624, -118.915) -> (137.62, -119.041)
  line L6775 (137.604, -118.633) -> (137.624, -118.915)
  line L6776 (136.476, -117.106) -> (136.722, -117.244)
  line L6777 (198.48, -116.971) -> (198.762, -116.956)
  line L6778 (137.145, -117.616) -> (137.313, -117.844)
  line L6779 (137.582, -119.321) -> (137.506, -119.593)
  line L6780 (136.36, -120.775) -> (136.091, -120.86)
  line L6781 (136.722, -117.244) -> (136.947, -117.415)
  line L6782 (198.762, -116.956) -> (199.043, -116.98)
  line L6783 (135.812, -120.906) -> (135.53, -120.913)
  line L6784 (194.096, -118.962) -> (194.259, -119.05)
  line L6785 (194.402, -119.168) -> (194.519, -119.312)
  line L6786 (136.615, -120.652) -> (136.36, -120.775)
  line L6787 (136.091, -120.86) -> (135.812, -120.906)
  line L6788 (133.625, -118.852) -> (133.654, -118.571)
  line L6789 (135.096, -116.986) -> (135.373, -116.931)
  line L6790 (133.654, -118.571) -> (133.722, -118.297)
  line L6791 (194.519, -119.312) -> (194.606, -119.475)
  line L6792 (198.203, -117.026) -> (198.48, -116.971)
  line L6793 (136.85, -120.496) -> (136.615, -120.652)
  line L6794 (135.53, -120.913) -> (135.249, -120.88)
  line L6795 (133.687, -119.413) -> (133.636, -119.135)
  line L6796 (194.259, -119.05) -> (194.402, -119.168)
  line L6797 (134.83, -117.08) -> (135.096, -116.986)
  line L6798 (134.579, -117.21) -> (134.83, -117.08)
  line L6799 (136.947, -117.415) -> (137.145, -117.616)
  line L6800 (133.776, -119.681) -> (133.687, -119.413)
  line L6801 (194.606, -119.475) -> (194.66, -119.653)
  line L6802 (194.678, -119.837) -> (194.677, -119.864)
  line L6803 (194.504, -120.385) -> (194.383, -120.525)
  line L6804 (194.237, -120.64) -> (194.071, -120.723)
  line L6805 (193.919, -118.907) -> (194.096, -118.962)
  line L6806 (133.97, -117.791) -> (134.145, -117.569)
  line L6807 (194.66, -119.653) -> (194.678, -119.837)
  line L6808 (133.828, -118.035) -> (133.97, -117.791)
  line L6809 (135.373, -116.931) -> (135.655, -116.915)
  line L6810 (194.383, -120.525) -> (194.237, -120.64)
  line L6811 (192.929, -120.352) -> (192.844, -120.187)
  line L6812 (134.349, -117.374) -> (134.579, -117.21)
  line L6813 (141.301, -119.128) -> (141.418, -119.272)
  line L6814 (135.655, -116.915) -> (135.937, -116.94)
  line L6815 (134.145, -117.569) -> (134.349, -117.374)
  line L6816 (193.708, -120.787) -> (193.524, -120.765)
  line L6817 (141.495, -120.184) -> (141.403, -120.345)
  line L6818 (193.207, -119.043) -> (193.372, -118.957)
  line L6819 (141.553, -120.008) -> (141.495, -120.184)
  line L6820 (192.844, -120.187) -> (192.793, -120.009)
  line L6821 (141.576, -119.824) -> (141.553, -120.008)
  line L6822 (192.854, -119.463) -> (192.944, -119.301)
  line L6823 (193.063, -119.159) -> (193.207, -119.043)
  line L6824 (141.577, -119.797) -> (141.576, -119.824)
  line L6825 (194.596, -120.224) -> (194.504, -120.385)
  line L6826 (140.995, -118.922) -> (141.158, -119.01)
  line L6827 (193.347, -120.708) -> (193.185, -120.618)
  line L6828 (141.158, -119.01) -> (141.301, -119.128)
  line L6829 (194.071, -120.723) -> (193.893, -120.773)
  line L6830 (193.893, -120.773) -> (193.708, -120.787)
  line L6831 (141.418, -119.272) -> (141.505, -119.435)
  line L6832 (140.97, -120.683) -> (140.792, -120.733)
  line L6833 (193.044, -120.497) -> (192.929, -120.352)
  line L6834 (193.185, -120.618) -> (193.044, -120.497)
  line L6835 (140.818, -118.867) -> (140.995, -118.922)
  line L6836 (315.542, -116.559) -> (315.788, -116.697)
  line L6837 (140.633, -118.847) -> (140.818, -118.867)
  line L6838 (133.722, -118.297) -> (133.828, -118.035)
  line L6839 (133.903, -119.933) -> (133.776, -119.681)
  line L6840 (141.403, -120.345) -> (141.282, -120.485)
  line L6841 (141.136, -120.599) -> (140.97, -120.683)
  line L6842 (193.734, -118.887) -> (193.919, -118.907)
  line L6843 (316.211, -117.069) -> (316.379, -117.297)
  line L6844 (140.085, -120.577) -> (139.943, -120.457)
  line L6845 (194.654, -120.048) -> (194.596, -120.224)
  line L6846 (133.636, -119.135) -> (133.625, -118.852)
  line L6847 (141.282, -120.485) -> (141.136, -120.599)
  line L6848 (192.798, -119.64) -> (192.854, -119.463)
  line L6849 (141.505, -119.435) -> (141.559, -119.613)
  line L6850 (140.607, -120.747) -> (140.423, -120.725)
  line L6851 (139.744, -120.147) -> (139.692, -119.969)
  line L6852 (192.793, -120.009) -> (192.778, -119.824)
  line L6853 (193.372, -118.957) -> (193.55, -118.904)
  line L6854 (194.677, -119.864) -> (194.654, -120.048)
  line L6855 (192.944, -119.301) -> (193.063, -119.159)
  line L6856 (141.559, -119.613) -> (141.577, -119.797)
  line L6857 (193.524, -120.765) -> (193.347, -120.708)
  line L6858 (193.55, -118.904) -> (193.734, -118.887)
  line L6859 (192.778, -119.824) -> (192.798, -119.64)
  line L6860 (140.423, -120.725) -> (140.246, -120.668)
  line L6861 (140.792, -120.733) -> (140.607, -120.747)
  line L6862 (139.692, -119.969) -> (139.677, -119.784)
  line L6863 (316.67, -118.086) -> (316.69, -118.368)
  line L6864 (316.649, -118.774) -> (316.572, -119.046)
  line L6865 (316.379, -117.297) -> (316.513, -117.545)
  line L6866 (139.677, -119.784) -> (139.698, -119.6)
  line L6867 (139.962, -119.119) -> (140.107, -119.002)
  line L6868 (140.449, -118.864) -> (140.633, -118.847)
  line L6869 (139.943, -120.457) -> (139.828, -120.312)
  line L6870 (140.107, -119.002) -> (140.271, -118.917)
  line L6871 (139.828, -120.312) -> (139.744, -120.147)
  line L6872 (139.754, -119.423) -> (139.843, -119.261)
  line L6873 (315.003, -116.393) -> (315.278, -116.457)
  line L6874 (313.211, -117.022) -> (313.415, -116.827)
  line L6875 (314.315, -120.333) -> (314.042, -120.26)
  line L6876 (313.321, -119.826) -> (313.129, -119.619)
  line L6877 (316.013, -116.868) -> (316.211, -117.069)
  line L6878 (312.702, -118.588) -> (312.691, -118.305)
  line L6879 (316.69, -118.368) -> (316.686, -118.494)
  line L6880 (314.042, -120.26) -> (313.782, -120.15)
  line L6881 (314.44, -116.384) -> (314.722, -116.368)
  line L6882 (314.722, -116.368) -> (315.003, -116.393)
  line L6883 (313.896, -116.533) -> (314.162, -116.439)
  line L6884 (139.698, -119.6) -> (139.754, -119.423)
  line L6885 (315.278, -116.457) -> (315.542, -116.559)
  line L6886 (316.572, -119.046) -> (316.458, -119.304)
  line L6887 (314.162, -116.439) -> (314.44, -116.384)
  line L6888 (313.645, -116.663) -> (313.896, -116.533)
  line L6889 (19.9771, -116.353) -> (20.2523, -116.417)
  line L6890 (312.894, -117.488) -> (313.036, -117.244)
  line L6891 (139.843, -119.261) -> (139.962, -119.119)
  line L6892 (140.246, -120.668) -> (140.085, -120.577)
  line L6893 (315.788, -116.697) -> (316.013, -116.868)
  line L6894 (313.129, -119.619) -> (312.969, -119.386)
  line L6895 (313.415, -116.827) -> (313.645, -116.663)
  line L6896 (316.513, -117.545) -> (316.611, -117.81)
  line L6897 (316.686, -118.494) -> (316.649, -118.774)
  line L6898 (312.842, -119.134) -> (312.753, -118.866)
  line L6899 (316.611, -117.81) -> (316.67, -118.086)
  line L6900 (140.271, -118.917) -> (140.449, -118.864)
  line L6901 (316.308, -119.544) -> (316.126, -119.76)
  line L6902 (21.1005, -119.72) -> (20.8901, -119.908)
  line L6903 (315.681, -120.105) -> (315.426, -120.228)
  line L6904 (316.126, -119.76) -> (315.916, -119.948)
  line L6905 (313.782, -120.15) -> (313.54, -120.004)
  line L6906 (315.157, -120.313) -> (314.878, -120.359)
  line L6907 (20.8901, -119.908) -> (20.6552, -120.065)
  line L6908 (20.4005, -120.188) -> (20.1312, -120.273)
  line L6909 (314.878, -120.359) -> (314.596, -120.366)
  line L6910 (21.4318, -119.264) -> (21.2823, -119.504)
  line L6911 (315.426, -120.228) -> (315.157, -120.313)
  line L6912 (313.036, -117.244) -> (313.211, -117.022)
  line L6913 (312.753, -118.866) -> (312.702, -118.588)
  line L6914 (312.72, -118.024) -> (312.788, -117.75)
  line L6915 (20.9869, -116.828) -> (21.1851, -117.029)
  line L6916 (21.5849, -117.77) -> (21.6443, -118.046)
  line L6917 (313.54, -120.004) -> (313.321, -119.826)
  line L6918 (312.691, -118.305) -> (312.72, -118.024)
  line L6919 (316.458, -119.304) -> (316.308, -119.544)
  line L6920 (312.788, -117.75) -> (312.894, -117.488)
  line L6921 (314.596, -120.366) -> (314.315, -120.333)
  line L6922 (312.969, -119.386) -> (312.842, -119.134)
  line L6923 (315.916, -119.948) -> (315.681, -120.105)
  line L6924 (310.464, -119.798) -> (310.343, -119.938)
  line L6925 (20.1312, -120.273) -> (19.8525, -120.319)
  line L6926 (19.1365, -116.399) -> (19.4136, -116.344)
  line L6927 (309.145, -120.03) -> (309.004, -119.91)
  line L6928 (18.87, -116.493) -> (19.1365, -116.399)
  line L6929 (18.0101, -117.204) -> (18.185, -116.982)
  line L6930 (20.5158, -116.518) -> (20.7623, -116.656)
  line L6931 (310.343, -119.938) -> (310.196, -120.052)
  line L6932 (309.852, -120.186) -> (309.668, -120.2)
  line L6933 (19.6957, -116.328) -> (19.9771, -116.353)
  line L6934 (309.307, -120.121) -> (309.145, -120.03)
  line L6935 (21.6643, -118.328) -> (21.6603, -118.454)
  line L6936 (18.2952, -119.786) -> (18.1034, -119.579)
  line L6937 (310.479, -118.725) -> (310.566, -118.888)
  line L6938 (309.668, -120.2) -> (309.483, -120.178)
  line L6939 (309.483, -120.178) -> (309.307, -120.121)
  line L6940 (17.9428, -119.346) -> (17.8165, -119.093)
  line L6941 (20.7623, -116.656) -> (20.9869, -116.828)
  line L6942 (21.2823, -119.504) -> (21.1005, -119.72)
  line L6943 (19.5701, -120.326) -> (19.2895, -120.293)
  line L6944 (21.1851, -117.029) -> (21.3529, -117.256)
  line L6945 (19.2895, -120.293) -> (19.0164, -120.22)
  line L6946 (17.7271, -118.825) -> (17.6763, -118.548)
  line L6947 (21.4871, -117.505) -> (21.5849, -117.77)
  line L6948 (19.0164, -120.22) -> (18.7563, -120.11)
  line L6949 (21.546, -119.006) -> (21.4318, -119.264)
  line L6950 (310.362, -118.581) -> (310.479, -118.725)
  line L6951 (17.8682, -117.448) -> (18.0101, -117.204)
  line L6952 (310.614, -119.461) -> (310.555, -119.637)
  line L6953 (20.6552, -120.065) -> (20.4005, -120.188)
  line L6954 (18.5143, -119.964) -> (18.2952, -119.786)
  line L6955 (18.7563, -120.11) -> (18.5143, -119.964)
  line L6956 (21.6443, -118.046) -> (21.6643, -118.328)
  line L6957 (17.7622, -117.71) -> (17.8682, -117.448)
  line L6958 (310.196, -120.052) -> (310.031, -120.136)
  line L6959 (310.637, -119.277) -> (310.614, -119.461)
  line L6960 (19.8525, -120.319) -> (19.5701, -120.326)
  line L6961 (21.3529, -117.256) -> (21.4871, -117.505)
  line L6962 (310.031, -120.136) -> (309.852, -120.186)
  line L6963 (17.8165, -119.093) -> (17.7271, -118.825)
  line L6964 (17.694, -117.984) -> (17.7622, -117.71)
  line L6965 (18.1034, -119.579) -> (17.9428, -119.346)
  line L6966 (21.6227, -118.734) -> (21.546, -119.006)
  line L6967 (17.6763, -118.548) -> (17.6653, -118.265)
  line L6968 (310.555, -119.637) -> (310.464, -119.798)
  line L6969 (21.6603, -118.454) -> (21.6227, -118.734)
  line L6970 (19.4136, -116.344) -> (19.6957, -116.328)
  line L6971 (17.6653, -118.265) -> (17.694, -117.984)
  line L6972 (20.2523, -116.417) -> (20.5158, -116.518)
  line L6973 (297.631, -101.083) -> (297.815, -101.103)
  line L6974 (297.446, -101.1) -> (297.631, -101.083)
  line L6975 (37.68, -101.993) -> (37.6797, -102.02)
  line L6976 (37.0982, -101.118) -> (37.2613, -101.206)
  line L6977 (36.9211, -101.063) -> (37.0982, -101.118)
  line L6978 (37.5213, -101.468) -> (37.6083, -101.631)
  line L6979 (37.6797, -102.02) -> (37.6564, -102.204)
  line L6980 (37.6619, -101.809) -> (37.68, -101.993)
  line L6981 (296.841, -101.497) -> (296.96, -101.355)
  line L6982 (298.134, -102.836) -> (297.968, -102.919)
  line L6983 (37.4041, -101.324) -> (37.5213, -101.468)
  line L6984 (37.6564, -102.204) -> (37.5979, -102.38)
  line L6985 (296.941, -102.693) -> (296.826, -102.548)
  line L6986 (296.695, -101.836) -> (296.751, -101.659)
  line L6987 (75.2673, -124.5) -> (75.1067, -124.267)
  line L6988 (75.1067, -124.267) -> (74.9804, -124.015)
  line L6989 (75.4591, -124.707) -> (75.2673, -124.5)
  line L6990 (77.141, -121.274) -> (77.4162, -121.338)
  line L6991 (77.2951, -125.194) -> (77.0164, -125.24)
  line L6992 (78.054, -124.83) -> (77.8191, -124.987)
  line L6993 (77.8191, -124.987) -> (77.5644, -125.109)
  line L6994 (257.558, -121.29) -> (257.839, -121.314)
  line L6995 (78.5957, -124.185) -> (78.4462, -124.425)
  line L6996 (75.6782, -124.886) -> (75.4591, -124.707)
  line L6997 (257.276, -121.305) -> (257.558, -121.29)
  line L6998 (78.651, -122.426) -> (78.7488, -122.691)
  line L6999 (78.7099, -123.927) -> (78.5957, -124.185)
  line L7000 (77.4162, -121.338) -> (77.6797, -121.44)
  line L7001 (78.5168, -122.178) -> (78.651, -122.426)
  line L7002 (78.8282, -123.249) -> (78.8242, -123.375)
  line L7003 (77.5644, -125.109) -> (77.2951, -125.194)
  line L7004 (76.5775, -121.265) -> (76.8596, -121.25)
  line L7005 (78.8242, -123.375) -> (78.7866, -123.655)
  line L7006 (78.7866, -123.655) -> (78.7099, -123.927)
  line L7007 (76.4534, -125.214) -> (76.1803, -125.141)
  line L7008 (77.6797, -121.44) -> (77.9262, -121.578)
  line L7009 (77.9262, -121.578) -> (78.1508, -121.749)
  line L7010 (252.867, -125.057) -> (252.688, -125.107)
  line L7011 (252.892, -123.296) -> (253.055, -123.384)
  line L7012 (76.7339, -125.247) -> (76.4534, -125.214)
  line L7013 (253.474, -124.171) -> (253.473, -124.198)
  line L7014 (74.8291, -123.186) -> (74.8579, -122.905)
  line L7015 (74.9804, -124.015) -> (74.891, -123.747)
  line L7016 (74.891, -123.747) -> (74.8402, -123.469)
  line L7017 (75.0321, -122.369) -> (75.174, -122.125)
  line L7018 (75.3489, -121.903) -> (75.5533, -121.708)
  line L7019 (252.715, -123.241) -> (252.892, -123.296)
  line L7020 (253.033, -124.974) -> (252.867, -125.057)
  line L7021 (252.504, -125.121) -> (252.32, -125.099)
  line L7022 (74.8579, -122.905) -> (74.9261, -122.631)
  line L7023 (74.8402, -123.469) -> (74.8291, -123.186)
  line L7024 (253.473, -124.198) -> (253.45, -124.382)
  line L7025 (75.7832, -121.544) -> (76.0339, -121.414)
  line L7026 (253.391, -124.558) -> (253.3, -124.719)
  line L7027 (76.0339, -121.414) -> (76.3004, -121.32)
  line L7028 (74.9261, -122.631) -> (75.0321, -122.369)